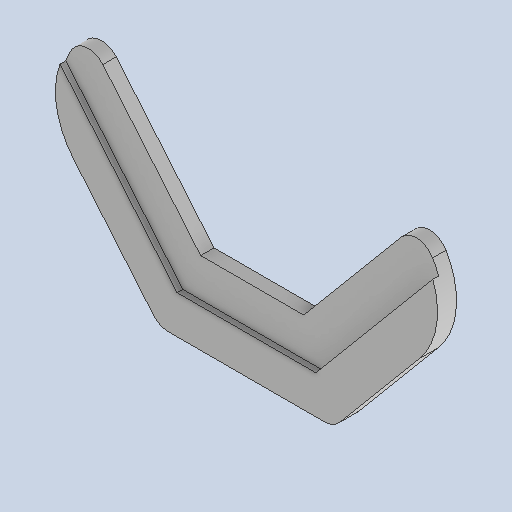
# Autodesk Inventor part: ДМС 045 держатель лотка
Saved by Autodesk Inventor 2024.2 (Build 282272000, 272)
## iProperties
Created: 2024-05-13
Part Number: ДМС 045 держатель лотка
Material: Generic
Document SubType Name: Modeling
Designer: admin
Density: 1 g/cm^3
Appearance: Default
Author: admin
Autodesk Inventor part; units mm, degrees
ref_plane "YZ Plane" through (0, 0, 0) normal (1, 0, 0) x (0, 1, 0)
ref_plane "XZ Plane" through (0, 0, 0) normal (0, 1, 0) x (-1, 0, 0)
ref_plane "XY Plane" through (0, 0, 0) normal (0, 0, 1) x (1, 0, 0)
sketch "Sketch1" plane through (0, 0, 0) normal (0, 1, 0) x (-1, 0, 0)
  line L0 (-27, 0) -> (27, 0)
  line L1 (-27, 0) -> (-85.737, 70)
  line L2 (85.737, 70) -> (27, 0)
  line L3 (90.6672, 13.6467) -> (45.6523, -40)
  line L4 (45.6523, -40) -> (-45.6523, -40)
  line L5 (-45.6523, -40) -> (-90.6672, 13.6467)
  line L6 (0, 0) -> (0, -40) construction
  arc A0 (90.6672, 13.6467) -> (85.737, 70) centre (60.0255, 39.3582) ccw
  arc A1 (-85.737, 70) -> (-90.6672, 13.6467) centre (-60.0255, 39.3582) ccw
  point P0 (0, 70)
  dimension "d1" = 54
  dimension "d3" = 40
  dimension "d5" = 40
  dimension "d16" = 130
  dimension "d17" = 70
  constraints: 14 end point, 4 point on circle, 2 centre point, 2 line through centre, 2 midpoint, 2 parallel, 2 tangent, 2 vertical alignment, 1 coincident, 1 equal length, 1 horizontal, 1 perpendicular, 1 other
  measures "d1" distance of L0.start L0.end
  measures "d3" distance between parallel lines of L4 L0
  measures "d5" distance between parallel lines of L3 L2
  measures "d16" angle of L0 L2
  measures "d17" distance from line of L0 L2.start
extrude "Extrusion1" add sketch "Sketch1" along normal blind 10
sketch "Sketch2" plane through (0, 0, 0) normal (0, -1, 0) x (1, 0, 0)
  line L0 (-27, 0) -> (27, 0) projected
  line L1 (-85.737, 70) -> (-27, 0) projected
  line L2 (-45.6523, -40) -> (-90.6672, 13.6467) construction
  line L3 (45.6523, -40) -> (-45.6523, -40) construction
  line L4 (90.6672, 13.6467) -> (45.6523, -40) construction
  line L5 (27, 0) -> (85.737, 70) projected
  line L6 (-97.6132, 53.039) -> (-36.3262, -20)
  line L7 (-36.3262, -20) -> (36.3262, -20)
  line L8 (36.3262, -20) -> (97.6132, 53.039)
  line L9 (-85.737, 70) -> (-27, 0) projected
  line L10 (27, 0) -> (85.737, 70) projected
  arc A0 (-85.737, 70) -> (-90.6672, 13.6467) centre (-60.0255, 39.3582) ccw projected
  arc A1 (90.6672, 13.6467) -> (85.737, 70) centre (60.0255, 39.3582) ccw projected
  point P0 (0, 0)
  dimension "d8" = 20
  dimension "d9" = 20
  dimension "d10" = 20
  constraints: 6 end point, 2 parallel, 2 point on circle, 1 horizontal
  measures "d8" distance between parallel lines of L7 L0
  measures "d9" distance between parallel lines of L1 L6
  measures "d10" distance between parallel lines of L5 L8
extrude "Extrusion2" cut sketch "Sketch2" against normal blind 3
fillet "Fillet1" radius 10 4 edges at (-85.737, 6.5, 70) (85.737, 6.5, 70) (-45.6523, 5, -40) (45.6523, 5, -40)
equation "\"d5\" = d3"
equation "\"d16\" = Лоток_угол"
equation "\"d9\" = d8"
equation "\"d10\" = d8"
equation "\"Лоток_угол\" = 130deg"
body "Solid1"
